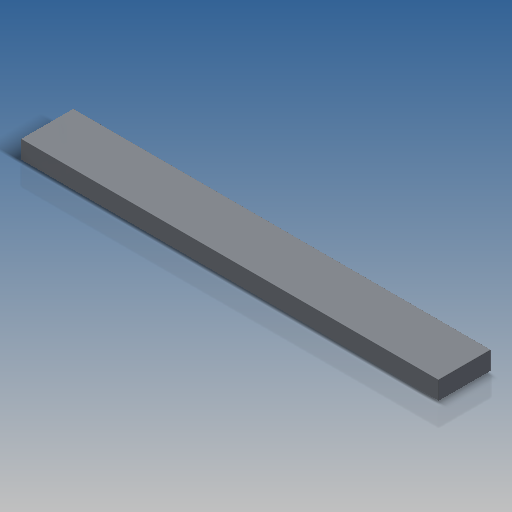
# Autodesk Inventor part: 4162-LtBluishGray
Saved by Autodesk Inventor 2018.3 (Build 223284000, 284)
## iProperties
Created: 2014-06-03
Part Number: 4162-LtBluishGray
Material: ABS Plastic
Document SubType Name: Modeling
Designer: D. Kohfeld
Density: 1.06 g/cm^3
Appearance: LtBluishGray
Mass: 1.31272 g
Surface Area: 17.9936 cm^2
Volume: 1.23842 cm^3
Author: D. Kohfeld
Autodesk Inventor part; units mm, degrees
ref_plane "YZ Plane" through (0, 0, 0) normal (1, 0, 0) x (0, 1, 0)
ref_plane "XZ Plane" through (0, 0, 0) normal (0, 1, 0) x (-1, 0, 0)
ref_plane "XY Plane" through (0, 0, 0) normal (0, 0, 1) x (1, 0, 0)
sketch "Sketch2" plane through (0, 0, 0) normal (0, 1, 0) x (-1, 0, 0)
  line L0 (-32, 4) -> (32, 4)
  line L1 (32, 4) -> (32, -4)
  line L2 (32, -4) -> (-32, -4)
  line L3 (-32, -4) -> (-32, 4)
  point P0 (0, 0)
  point P1 (0, 4)
  point P2 (-32, 0)
  dimension "d0" = 64
  dimension "d1" = 8
  constraints: 8 end point, 2 midpoint, 2 parallel, 1 horizontal, 1 horizontal alignment, 1 perpendicular, 1 vertical alignment
  measures "d0" distance of L1.end L2.end
  measures "d1" distance of L2.end L0.start
extrude "Extrusion1" add sketch "Sketch2" along normal blind 3.2
sketch "Sketch3" plane through (0, 0, 0) normal (0, -1, 0) x (1, 0, 0)
  line L0 (32, 4) -> (-32, 4) projected
  line L1 (-32, 4) -> (-32, -4) projected
  line L2 (-30.4, 2.4) -> (30.4, 2.4)
  line L3 (30.4, 2.4) -> (30.4, -2.4)
  line L4 (30.4, -2.4) -> (-30.4, -2.4)
  line L5 (-30.4, -2.4) -> (-30.4, 2.4)
  circle A0 centre (-24, 4) radius 3.2569
  circle A1 centre (-24, 4) radius 2.4
  line L6 (-32, -4) -> (32, -4) projected
  circle A2 centre (0, 0) radius 1.6
  line L7 (32, -4) -> (32, 4) projected
  line L8 (-20, 0) -> (-12, 0) construction
  line L9 (-12, 0) -> (-4, 0) construction
  line L10 (4, 0) -> (12, 0) construction
  line L11 (12, 0) -> (20, 0) construction
  line L12 (-4, 0) -> (4, 0) construction
  line L13 (-28, 0) -> (-20, 0) construction
  line L14 (20, 0) -> (28, 0) construction
  line L15 (-31.6, 3.6) -> (31.6, 3.6)
  line L16 (31.6, 3.6) -> (31.6, -3.6)
  line L17 (31.6, -3.6) -> (-31.6, -3.6)
  line L18 (-31.6, -3.6) -> (-31.6, 3.6)
  point P0 (-30.4, 0)
  point P1 (0, 2.4)
  point P2 (0, 3.6)
  point P3 (-31.6, 0)
  dimension "d8" = 1.6
  dimension "d60" = 6.5137
  dimension "d61" = 4.8
  dimension "d62" = 1.6
  dimension "d75" = 8
  dimension "d76" = 8
  dimension "d86" = 3.2
  dimension "d93" = 8
  dimension "d99" = 0.4
  dimension "d100" = 0.4
  constraints: 30 end point, 10 equal length, 6 collinear, 5 midpoint, 3 centre point, 3 coincident, 3 perpendicular, 2 horizontal, 2 horizontal alignment, 2 vertical alignment
  measures "d8" distance between parallel lines of L1 L5
  measures "d60" diameter of A0
  measures "d61" diameter of A1
  measures "d62" distance between parallel lines of L0 L2
  measures "d75" distance from line of A0.centre L1
  measures "d76" distance from line of A0.centre L6
  measures "d86" diameter of A2
  measures "d93" distance of L9.end L10.start
  measures "d99" distance between parallel lines of L0 L15
  measures "d100" distance between parallel lines of L1 L18
extrude "Extrusion2" cut sketch "Sketch3" against normal blind 1.6 contours A0 L2 A1 | L2 L3 L4 L5 A0 | A1 L2 | A2
extrude "Extrusion7" cut sketch "Sketch3" against normal blind 0.4 contours L7 L6 L1 L0 A0 L15 L18 L17 L16 | A0 L15 A1 L0 | A1 L15 L0 | L0 A1 L15 A0
extrude "Extrusion6" add sketch "Sketch3" against normal up to next contours A2
pattern_linear "Rectangular Pattern3" count 7 spacing 8 along (-1, 0, 0) of "Extrusion6" first direction both ways yes
fillet "Fillet1" radius 0.1 8 edges at (-32, 1.8, 4) (0, 3.2, 4) (-32, 3.2, 0) (32, 1.8, 4) (32, 3.2, 0) (0, 3.2, -4) (32, 1.8, -4) (-32, 1.8, -4)
equation "\"d4\" = 0.333333 * lh"
equation "\"d8\" = d62"
equation "\"d60\" = tubeod"
equation "\"d61\" = kd"
equation "\"d62\" = wall"
equation "\"d75\" = lu"
equation "\"d76\" = d75"
equation "\"d86\" = pd"
equation "\"d93\" = lu"
equation "\"d99\" = gw"
equation "\"d100\" = gw"
equation "\"d11\" = 0.333333 * lh - topthk"
equation "\"d101\" = gh"
equation "\"d91\" = lu"
equation "\"d22\" = lf"
equation "\"lh\" = 9.6"
equation "\"tubeod\" = 6.513708"
equation "\"kd\" = 4.8"
equation "\"wall\" = 1.6"
equation "\"lu\" = 8"
equation "\"pd\" = 3.2"
equation "\"gw\" = 0.4"
equation "\"topthk\" = 1.6"
equation "\"gh\" = 0.4"
equation "\"lf\" = 0.1"
body "Solid1"
